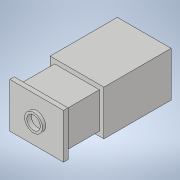
# Autodesk Inventor part: Micro Gearmotors
Saved by Autodesk Inventor 2020 (Build 240168000, 168)
## iProperties
Created: 2020-02-04
Part Number: Micro Gearmotors
Material: Типовые
Document SubType Name: Modeling
Designer: ШП
Density: 1 g/cm^3
Appearance: По умолчанию
Author: ШП
Autodesk Inventor part; units mm, degrees
ref_plane "YZ Plane" through (0, 0, 0) normal (1, 0, 0) x (0, 1, 0)
ref_plane "XZ Plane" through (0, 0, 0) normal (0, 1, 0) x (-1, 0, 0)
ref_plane "XY Plane" through (0, 0, 0) normal (0, 0, 1) x (1, 0, 0)
sketch "Эскиз2" plane through (0, 0, 0) normal (0, 0, 1) x (1, 0, 0)
  line L0 (0, 0) -> (12, 0)
  line L1 (12, 0) -> (12, 10)
  line L2 (12, 10) -> (0, 10)
  line L3 (0, 10) -> (0, 0)
  line L4 (-15.2128, 15.4518) -> (-15.9082, 15.4518)
  line L5 (-15.9082, 15.4518) -> (-15.9082, 15.4083)
  line L6 (-15.9082, 15.4083) -> (-15.2128, 15.4083)
  line L7 (-15.2128, 15.4083) -> (-15.2128, 15.4518)
  dimension "d0" = 12
  dimension "d1" = 10
  constraints: 16 end point, 4 parallel, 2 horizontal, 2 perpendicular
  measures "d0" distance of L2.end L1.end
  measures "d1" distance of L1.end L0.end
extrude "Выдавливание1" add sketch "Эскиз2" along normal blind 1 contours L3 L2 L1 L0
sketch "Эскиз3" plane through (0, 0, 1) normal (0, 0, 1) x (1, 0, 0)
  line L0 (0, 10) -> (0, 0) projected
  line L1 (0, 5) -> (12, 5)
  line L2 (12, 0) -> (12, 10) projected
  circle A0 centre (6, 5) radius 2
  dimension "d4" = 4
  constraints: 3 midpoint, 2 end point, 1 centre point
  measures "d4" diameter of A0
extrude "Выдавливание2" add sketch "Эскиз3" along normal blind 0.7
sketch "Эскиз5" plane through (0, 0, 0) normal (0, 0, -1) x (-1, 0, 0)
  line L0 (-12, 10) -> (0, 10) projected
  line L1 (0, 10) -> (0, 0) projected
  line L2 (-12, 10) -> (0, 10)
  line L3 (0, 10) -> (0, 0)
  line L4 (0, 0) -> (-12, 0)
  line L5 (-12, 0) -> (-12, 10)
  line L6 (-12, 10) -> (-11, 10)
  line L7 (-11, 10) -> (-11, 9)
  line L8 (-11, 9) -> (-1, 9)
  line L9 (-1, 9) -> (-1, 1)
  line L10 (-1, 1) -> (-11, 1)
  line L11 (-11, 1) -> (-11, 9)
  dimension "d22" = 1
  dimension "d23" = 1
  dimension "d24" = 10
  dimension "d25" = 8
  dimension "d26" = 12
  dimension "d27" = 10
  constraints: 20 end point, 4 parallel, 3 perpendicular, 2 horizontal, 1 point on line
  measures "d22" distance of L0.start L6.end
  measures "d23" distance of L6.end L7.end
  measures "d24" distance of L9.end L10.end
  measures "d25" distance of L8.end L9.end
  measures "d26" distance of L0.start L0.end
  measures "d27" distance of L0.end L1.end
extrude "Выдавливание4" add sketch "Эскиз5" along normal blind 8 contours L8 L9 L10 L11
sketch "Эскиз6" plane through (0, 0, -8) normal (0, 0, -1) x (-1, 0, 0)
  line L0 (-12, 10) -> (0, 10) projected
  line L1 (0, 10) -> (0, 0) projected
  line L2 (-12, 10) -> (0, 10)
  line L3 (0, 10) -> (0, 0)
  line L4 (0, 0) -> (-12, 0)
  line L5 (-12, 0) -> (-12, 10)
  constraints: 8 end point, 2 parallel, 1 horizontal, 1 perpendicular
extrude "Выдавливание5" add sketch "Эскиз6" along normal blind 15
sketch "Эскиз11" plane through (6, 5, 1.7) normal (0, 0, 1) x (1, 0, 0)
  circle A0 centre (0, 0) radius 1.5
  point P0 (-6, -5)
  dimension "d32" = 3
  constraints: 1 centre point
  measures "d32" diameter of A0
extrude "Выдавливание9" cut sketch "Эскиз11" against normal blind 1
sketch "Эскиз8" plane through (0, 0, -23) normal (0, 0, -1) x (-1, 0, 0)
  circle A0 centre (-6, 5) radius 2 projected
  circle A1 centre (-6, 5) radius 2.5
  point P0 (0, 0)
  dimension "d15" = 5
  constraints: 1 centre point, 1 coincident
  measures "d15" diameter of A1
extrude "Выдавливание6" add sketch "Эскиз8" along normal blind 0.5 contours A0
equation "\"d22\" = -0.5 * d24 + 0.5 * d26"
equation "\"d23\" = -0.5 * d25 + 0.5 * d27"
